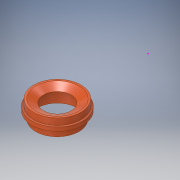
# Autodesk Inventor part: part 2 cap of Phenolic Master Sketch
Saved by Autodesk Inventor 2017 (Build 210142000, 142)
## iProperties
Created: 2016-07-25
Part Number: part 2 cap of Phenolic Master Sketch
Material: Phenolic Resin
Document SubType Name: Modeling
Designer: Jared
Density: 1.38 g/cm^3
Appearance: Smooth - Light Orange
Author: Jared
Autodesk Inventor part; units mm, degrees
sketch "Sketch2" plane through (0, 0, 0) normal (0, 1, 0) x (-1, 0, 0)
  line L0 (0, -114.5678) -> (107.9834, -114.5678)
  line L1 (107.9834, -114.5678) -> (107.9834, 108.3126)
  line L2 (107.9834, 108.3126) -> (0, 108.3126)
  line L3 (0, 108.3126) -> (0, -114.5678)
  point P0 (0, 0)
  constraints: 8 end point, 2 parallel, 1 horizontal, 1 perpendicular
extrude "Extrusion1" [suppressed]
ref_plane "Work Plane4" through (0, -133.7486, -73.152) normal (-1, 0, 0) x (0, 0, 1)
sketch "Sketch3" plane through (0, -133.7486, -73.152) normal (-1, 0, 0) x (0, 0, 1)
  line L0 (6.35, 143.6785) -> (6.35, 121.0486)
  line L1 (6.35, 121.0486) -> (6.35, 95.6486)
  line L2 (0, 95.6486) -> (6.35, 95.6486)
  line L3 (0, 121.0486) -> (-13.208, 121.0486)
  line L4 (-13.208, 121.0486) -> (-13.208, 133.7486) projected
  line L5 (-13.208, 121.0486) -> (-13.208, 133.7486)
  line L6 (-13.208, 133.7486) -> (-6.858, 133.7486)
  line L7 (-6.858, 133.7486) -> (-6.858, 156.1875)
  line L8 (-0.508, 156.1875) -> (26.3176, 143.6785) projected
  line L9 (-6.858, 156.1875) -> (-0.508, 156.1875)
  line L10 (-0.508, 156.1875) -> (26.3176, 143.6785)
  line L11 (12.7, 143.6785) -> (26.3176, 143.6785)
  line L12 (6.35, 143.6785) -> (12.7, 143.6785)
  line L13 (314.1117, 153.1152) -> (314.1117, 130.4853)
  line L14 (314.1117, 130.4853) -> (314.1117, 105.0853)
  line L15 (307.7617, 105.0853) -> (314.1117, 105.0853)
  line L16 (307.7617, 130.4853) -> (294.5537, 130.4853)
  line L17 (294.5537, 130.4853) -> (294.5537, 143.1853)
  line L18 (294.5537, 143.1853) -> (300.9037, 143.1853)
  line L19 (300.9037, 143.1853) -> (300.9037, 165.6242)
  line L20 (307.2537, 165.6242) -> (334.0793, 153.1152)
  line L21 (300.9037, 165.6242) -> (307.2537, 165.6242)
  line L22 (320.4617, 153.1152) -> (334.0793, 153.1152)
  line L23 (314.1117, 153.1152) -> (320.4617, 153.1152)
  line L24 (334.0793, 153.1152) -> (380.9169, 153.1152) construction
  line L25 (380.9169, 153.1152) -> (380.9169, 203.9215) construction
  line L26 (307.7617, 130.4853) -> (307.7617, 105.0853)
  line L27 (0, 121.0486) -> (0, 95.6486)
  line L28 (0, 0) -> (0, 121.0486) projected
  point P0 (73.152, 133.7486)
  dimension "d32" = 6.35
  dimension "d34" = 6.35
  dimension "d35" = 46.8376
  constraints: 52 end point, 4 vertical, 3 collinear, 3 horizontal
  measures "d32" distance of L4.end L6.end
  measures "d34" distance of L17.end L18.end
  measures "d35" distance of L20.end L24.end
revolve "Revolution3" add sketch "Sketch3" angle 360 about axis through (0, 19.3666, 307.7649) along (0, 1, 0) contours L13 L14 L15 L26 L16 L17 L18 L19 L21 L20 L22 L23
ref_plane "Work Plane3" through (0, -133.7486, -73.152) normal (-1, 0, 0) x (0, 0, 1)
sketch "Sketch6" plane through (0, -133.7486, -73.152) normal (-1, 0, 0) x (0, 0, 1)
  line L0 (0, 121.0486) -> (0, 95.6486)
  line L1 (0, 95.6486) -> (6.35, 95.6486)
  line L2 (0, 121.0486) -> (-13.208, 121.0486)
  line L3 (-13.208, 121.0486) -> (-13.208, 133.7486) projected
  line L4 (-13.208, 121.0486) -> (-13.208, 133.7486)
  line L5 (-13.208, 133.7486) -> (-6.858, 133.7486)
  line L6 (-6.858, 133.7486) -> (-6.858, 156.1875)
  line L7 (-0.508, 156.1875) -> (26.3176, 143.6785) projected
  line L8 (-6.858, 156.1875) -> (-0.508, 156.1875)
  line L9 (-0.508, 156.1875) -> (26.3176, 143.6785)
  line L10 (6.35, 95.6486) -> (6.35, 143.68)
  line L11 (6.35, 143.68) -> (26.3176, 143.6785)
  line L12 (26.3176, 143.6785) -> (92.5608, 143.6785) construction
  line L13 (73.152, 133.7486) -> (73.152, 183.9478) construction
  line L14 (119.9864, 143.6785) -> (26.3176, 143.6785) construction
  line L15 (26.3176, 143.6785) -> (73.152, 143.6785) construction
  dimension "d37" = 25.4
  dimension "d38" = 6.35
  dimension "d39" = 6.35
  dimension "d40" = 48.0314
  constraints: 26 end point, 2 collinear, 2 vertical, 1 midpoint, 1 perpendicular
  measures "d37" distance of L0.start L0.end
  measures "d38" distance of L0.end L1.end
  measures "d39" distance of L3.end L5.end
  measures "d40" distance of L1.end L10.end
revolve "Revolution4" cut sketch "Sketch6" angle 360 about axis through (0, 0, 0) along (0, 1, 0)
ref_plane "Work Plane2" through (0, 9.93, 0) normal (0, -1, 0) x (1, 0, 0)
sketch "Sketch7" plane through (0, 9.93, 0) normal (0, -1, 0) x (1, 0, 0)
  point P0 (0, 0)
ref_plane "Work Plane1" through (0, 9.93, 0) normal (0, -1, 0) x (1, 0, 0)
sketch "Sketch8" plane through (0, 9.93, 0) normal (0, -1, 0) x (1, 0, 0)
  point P0 (0, 0)
ref_plane "Work Plane5" through (0, 9.93, 0) normal (0, -1, 0) x (1, 0, 0)
sketch "Sketch9" plane through (0, 9.93, 0) normal (0, -1, 0) x (1, 0, 0)
  circle A0 centre (0, 0) radius 60.7129
  constraints: 1 centre point, 1 coincident
extrude "Extrusion2" cut sketch "Sketch9" along normal mid plane 25.4
body "Solid2"
